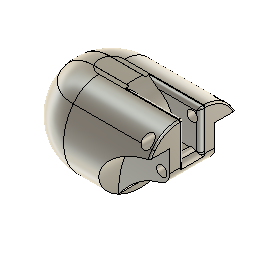
piece_4 (Autodesk Fusion 360 design; units mm, degrees)
Autodesk Fusion 360 part; units mm, degrees
sketch "Esboço1" plane through (0, 0, 0) normal (1, 0, 0) x (0, 1, 0)
  circle A0 centre (0, 0) radius 15
  dimension "d1" = 30
  constraint coincident A0.centre origin
  measures "d1" diameter of A0
extrude "Extrusão1" add sketch "Esboço1" along normal blind 40 makes body 1
fillet "Arredondamento1" radius 15 1 faces at (0, 3.8315, 5.6199) on bodies 1
sketch "Esboço2" plane through (40, 0, 0) normal (1, 0, 0) x (0, 1, 0)
  circle A0 centre (0, 0) radius 15
  line L0 (7.5, -12.9904) -> (-7.5, -12.9904)
  line L1 (-7.5, -12.9904) -> (-7.5, -7.9904)
  line L2 (-7.5, -7.9904) -> (7.5, -7.9904)
  line L3 (7.5, -7.9904) -> (7.5, -12.9904)
  line L4 (-7.5, -7.9904) -> (-15, -7.9904)
  line L5 (-15, -7.9904) -> (-15, -12.9904)
  line L6 (-15, -12.9904) -> (-7.5, -12.9904)
  line L7 (7.5, -7.9904) -> (15, -7.9904)
  line L8 (15, -7.9904) -> (15, -12.9904)
  line L9 (15, -12.9904) -> (7.5, -12.9904)
  dimension "d6" = 15
  dimension "d7" = 5
  dimension "d8" = 15
  constraint coincident A0 L0.start
  constraint coincident A0 L0.end
  constraint horizontal L0
  constraint perpendicular L0 L1
  constraint perpendicular L1 L2
  constraint perpendicular L1 L4
  constraint perpendicular L4 L5
  constraint perpendicular L1 L6
  constraint perpendicular L3 L7
  constraint perpendicular L2 L8
  constraint perpendicular L3 L9
  measures "d6" distance of L0.start L0.end
  measures "d7" distance of L0.end L1.end
  measures "d8" distance of L1.end L2.end
extrude "Extrusão2" cut sketch "Esboço2" against normal blind 5 contours A0 L1 L4 | A0 L3 L7 bodies 1
ref_plane "Plano de trabalho1" through (0, -16, 0) normal (0, 1, 0) x (0, 0, 1)
sketch "Esboço3" plane through (0, -16, 0) normal (0, 1, 0) x (1, 0, 0)
  spline S0 degree 5 poles (16, 15) (15.9441, 13.8206) (15.8879, 11.5162) (15.9712, 8.2226) (16.4224, 4.1625) (17.5919, -0.3229) (19.4201, -4.1668) (21.9593, -7.3182) (25.2357, -9.7517) (29.217, -11.4985) (33.8488, -12.6118) (38.0314, -13.0377) (41.4196, -13.1125) (43.7882, -13.0553) (45, -13) knots 0 0 0 0 0 0 0.1 0.2 0.3 0.4 0.5 0.6 0.7 0.8 0.9 1 1 1 1 1 1
  line L0 (16, 15) -> (45, 15)
  line L1 (45, 15) -> (45, -13)
  point P0 (22, -7)
  constraint horizontal L0
  constraint perpendicular L0 L1
extrude "Extrusão3" cut sketch "Esboço3" along normal blind 9 bodies 1
mirror "Espelhar1" about plane through (0, 0, 0) normal (0, 1, 0) of "Extrusão3"
sketch "Esboço4" plane through (0, -7, 0) normal (0, -1, 0) x (1, 0, 0)
  line L0 (15.9414, -13.2665) -> (40, -13.2665)
  spline S0 degree 5 poles (15.9414, -13.2665) (15.9255, -12.4614) (15.9203, -10.5419) (16.0411, -7.6201) (16.4922, -3.8951) (17.5919, 0.3229) (19.4201, 4.1668) (21.9593, 7.3182) (25.2357, 9.7517) (29.217, 11.4985) (33.0533, 12.4206) (36.2575, 12.8334) (38.5721, 12.9877) (39.8423, 13.0344) (40, 13.0397) knots 0.029806 0.029806 0.029806 0.029806 0.029806 0.029806 0.1 0.2 0.3 0.4 0.5 0.6 0.7 0.8 0.9 0.914124 0.914124 0.914124 0.914124 0.914124 0.914124
  circle A0 centre (37.5, -10.2665) radius 1.6
  line L1 (40, -13.2665) -> (40, 13.0397)
  dimension "d16" = 3.2
  dimension "d18" = 3
  dimension "d53" = 2.5
  measures "d16" diameter of A0
  measures "d18" distance of L0 A0.centre
  measures "d53" distance of A0.centre L1
extrude "Extrusão4" cut sketch "Esboço4" against normal blind 14 contours A0 bodies 1
sketch "Esboço5" plane through (40, 0, 0) normal (1, 0, 0) x (0, 1, 0)
  arc A0 (7.4139, 13.0397) -> (-7.4139, 13.0397) centre (0, 0) ccw
  line L0 (-2.5, 14.7902) -> (2.5, 14.7902)
  line L1 (2.5, 14.7902) -> (2.5, 1)
  line L2 (2.5, 1) -> (-2.5, 1)
  line L3 (-2.5, 1) -> (-2.5, 14.7902)
  line L4 (7, -13.2665) -> (7, 13.0397)
  line L5 (7, 13.0397) -> (7.4139, 13.0397)
  line L6 (-7.4139, 13.0397) -> (-7, 13.0397)
  line L7 (-7, 13.0397) -> (-7, -13.2665)
  arc A1 (-7, -13.2665) -> (7, -13.2665) centre (0, 0) ccw
  dimension "d21" = 5
  dimension "d22" = 2.5
  constraint horizontal L0
  constraint vertical L1
  constraint horizontal L2
  constraint vertical L3
  constraint coincident A0 L0.start
  measures "d21" distance of L0.start L0.end
  measures "d22" distance of A0.centre L3
extrude "Extrusão5" cut sketch "Esboço5" against normal blind 8 contours A0 L0 | L0 L1 L2 L3 bodies 1
sketch "Esboço6" plane through (0, 2.5, 0) normal (0, -1, 0) x (1, 0, 0)
  line L0 (40, 1) -> (40, 14.7902)
  line L1 (40, 14.7902) -> (32, 14.7902)
  line L2 (32, 14.7902) -> (32, 1)
  line L3 (32, 1) -> (40, 1)
  circle A0 centre (37.5, 9.7342) radius 1.6
  dimension "d25" = 3.2
  dimension "d26" = 2.5
  dimension "d27" = 5.056
  measures "d25" diameter of A0
  measures "d26" distance of L0 A0.centre
  measures "d27" distance of L1 A0.centre
extrude "Extrusão6" cut sketch "Esboço6" against normal blind 14 contours A0 bodies 1
extrude "Extrusão7" cut sketch "Esboço6" along normal blind 22 contours A0 bodies 1
copy_body "Corpo -> Componente1" bodies 1 removing the originals makes body 2 in component "Component'"
sketch "Esboço7" plane through (40, 0, 0) normal (1, 0, 0) x (0, 1, 0)
  line L0 (2.5, 14.7902) -> (2.5, 1)
  line L1 (2.5, 1) -> (-2.5, 1)
  line L2 (-2.5, 1) -> (-2.5, 14.7902)
  arc A0 (-2.5, 14.7902) -> (-7.4139, 13.0397) centre (0, 0) ccw
  line L3 (-7.4139, 13.0397) -> (-7, 13.0397)
  line L4 (-7, 13.0397) -> (-7, -13.2665)
  arc A1 (-7, -13.2665) -> (7, -13.2665) centre (0, 0) ccw
  line L5 (7, -13.2665) -> (7, 13.0397)
  line L6 (7, 13.0397) -> (7.4139, 13.0397)
  arc A2 (7.4139, 13.0397) -> (2.5, 14.7902) centre (0, 0) ccw
  line L7 (-7.4139, 13.0397) -> (7.4139, 13.0397)
  constraint coincident A0.end L3.start
  constraint coincident L6.end A2.start
extrude "Extrusão1'" cut sketch "Esboço7" against normal blind 8 contours L0 L6 A2 L7 | L2 A0 L3 L7 bodies 2 in component "Component'"
sketch "Esboço8" plane through (32, 0, 0) normal (1, 0, 0) x (0, 1, 0)
  arc A0 (7.4139, 13.0397) -> (-7.4139, 13.0397) centre (0, 0) ccw
  line L0 (-7.4139, 13.0397) -> (-2.5, 13.0397)
  line L1 (-2.5, 13.0397) -> (-2.5, 1)
  line L2 (-2.5, 1) -> (2.5, 1)
  line L3 (2.5, 1) -> (2.5, 13.0397)
  line L4 (2.5, 13.0397) -> (7.4139, 13.0397)
  line L5 (-2.5, 13.0397) -> (2.5, 13.0397)
  constraint coincident L0.end L1.start
  constraint coincident L3.end L4.start
fillet "Arredondamento5" radius 2 1 edges at (40, 0, 1) on bodies 2 in component "Component'"
sketch "Esboço9" plane through (0, -7, 0) normal (0, -1, 0) x (1, 0, 0)
  circle A0 centre (37.5, -10.2665) radius 1.6
  circle A1 centre (37.5, 9.7342) radius 1.6
  spline S0 degree 5 poles (15.9414, -13.2665) (15.9255, -12.4614) (15.9203, -10.5419) (16.0411, -7.6201) (16.4922, -3.8951) (17.5919, 0.3229) (19.4201, 4.1668) (21.9593, 7.3182) (25.2357, 9.7517) (29.217, 11.4985) (33.0533, 12.4206) (36.2575, 12.8334) (38.5721, 12.9877) (39.8423, 13.0344) (40, 13.0397) knots 0.029806 0.029806 0.029806 0.029806 0.029806 0.029806 0.1 0.2 0.3 0.4 0.5 0.6 0.7 0.8 0.9 0.914124 0.914124 0.914124 0.914124 0.914124 0.914124
  line L0 (15.9414, -13.2665) -> (40, -13.2665)
  spline S1 degree 5 poles (15.9414, -13.2665) (15.9568, -12.2565) (16.028, -10.2751) (16.2558, -7.4185) (16.8058, -3.8447) (17.9316, 0.204) (19.536, 3.7958) (21.6598, 6.8918) (24.3281, 9.4678) (27.5235, 11.5408) (31.2077, 13.147) (34.5148, 14.0885) (37.1849, 14.6135) (39.0478, 14.8844) (40, 15) knots 0 0 0 0 0 0 0.1 0.2 0.3 0.4 0.5 0.6 0.7 0.8 0.9 1 1 1 1 1 1
  line L1 (40, 15) -> (40, -13.2665)
  line L2 (40, -13.2665) -> (15.9414, -13.2665)
  line L3 (40, -13.2665) -> (40, 13.0397)
  point P0 (22, 7)
  constraint coincident S0.start L0.start
  constraint coincident S0 P0
  constraint perpendicular L0 L1
  constraint perpendicular L1 L2
extrude "Extrusão3'" cut sketch "Esboço9" along normal blind 14 contours S0 L0 S1 L1 L2 L3 | S0 S1 L1 bodies 2 in component "Component'"
mirror "Espelhar1'" about plane through (0, 0, 0) normal (0, 1, 0) of "Extrusão3'" in component "Component'"
sketch "Esboço10" plane through (0, -7, 0) normal (0, -1, 0) x (1, 0, 0)
  circle A0 centre (37.5, 9.7342) radius 1.6
  circle A1 centre (37.5, -10.2665) radius 1.6
  spline S0 degree 5 poles (15.9414, -13.2665) (15.9255, -12.4614) (15.9203, -10.5419) (16.0411, -7.6201) (16.4922, -3.8951) (17.5804, 0.2785) (19.0183, 3.3218) (20.4014, 5.2937) (21.4541, 6.4625) (22, 7) knots 0.029806 0.029806 0.029806 0.029806 0.029806 0.029806 0.1 0.2 0.3 0.4 0.495047 0.495047 0.495047 0.495047 0.495047 0.495047
  line L0 (15.9414, -13.2665) -> (40, -13.2665)
  spline S1 degree 5 poles (22, 7) (22.4471, 7.5113) (23.4297, 8.536) (25.0754, 9.9523) (27.0517, 11.2242) (29.2603, 12.2744) (30.9211, 12.9094) (31.8461, 13.2223) (31.9791, 13.2665) knots 0.508452 0.508452 0.508452 0.508452 0.508452 0.508452 0.6 0.7 0.8 0.816707 0.816707 0.816707 0.816707 0.816707 0.816707
  spline S2 degree 5 poles (33, -16) (32.9845, -15.3571) (32.9747, -14.0983) (33.0237, -12.2917) (33.2186, -10.0487) (33.6935, -7.5407) (34.4229, -5.3583) (35.4317, -3.5334) (36.7405, -2.0922) (38.3487, -1.034) (40.2384, -0.336) (41.9594, -0.0452) (43.3607, 0.0315) (44.3432, 0.0208) (44.8465, 0) knots 0 0 0 0 0 0 0.1 0.2 0.3 0.4 0.5 0.6 0.7 0.8 0.9 1 1 1 1 1 1
  line L1 (33, -16) -> (44.8465, -16)
  line L2 (44.8465, -16) -> (44.8465, 0)
  line L3 (40, -13.2665) -> (40, 13.0397)
  line L4 (40, 13.0397) -> (32, 13.0397)
  line L5 (32, 13.0397) -> (32, 13.2665)
  line L6 (32, 13.2665) -> (31.9791, 13.2665)
  point P0 (36, -3)
  constraint perpendicular L1 L2
sketch "Esboço11" plane through (40, 0, 0) normal (1, 0, 0) x (0, 1, 0)
  line L0 (-2.5, -1) -> (-2.5, 13.0397)
  line L1 (-2.5, 13.0397) -> (-7, 13.0397)
  line L2 (-7, 13.0397) -> (-7, -13.2665)
  arc A0 (-7, -13.2665) -> (7, -13.2665) centre (0, 0) ccw
  line L3 (7, -13.2665) -> (7, 13.0397)
  line L4 (2.5, 13.0397) -> (2.5, -1)
  line L5 (2.5, -1) -> (-2.5, -1)
  circle A1 centre (0, 0) radius 15
  line L6 (7, 13.0397) -> (2.5, 13.0397)
  line L7 (-2.5, 13.0397) -> (2.5, 13.0397)
  dimension "d62" = 30
  constraint concentric A0 A1
  constraint coincident L0.end L1.start
  constraint coincident L4.start L6.end
  measures "d62" diameter of A1
extrude "Extrusão5'" add sketch "Esboço11" against normal blind 25 contours L1 L2 L3 A1 L6 L7 bodies 2 in component "Component'"
sketch "Esboço12" plane through (0, -16, 0) normal (0, 1, 0) x (1, 0, 0)
  spline S0 degree 5 poles (24, 15) (23.9922, 14.2256) (24.0046, 12.7054) (24.1071, 10.5108) (24.4146, 7.7588) (25.1035, 4.6295) (26.1261, 1.8405) (27.5131, -0.5768) (29.2866, -2.5998) (31.4398, -4.2355) (33.9474, -5.5097) (36.2155, -6.2618) (38.0549, -6.6849) (39.3415, -6.9052) (40, -7) knots 0 0 0 0 0 0 0.1 0.2 0.3 0.4 0.5 0.6 0.7 0.8 0.9 1 1 1 1 1 1
  line L0 (24, 15) -> (40, 15)
  line L1 (40, 15) -> (40, -7)
  point P0 (28, -1)
  constraint horizontal L0
  constraint perpendicular L0 L1
extrude "Extrusão6'" cut sketch "Esboço12" along normal blind 9 bodies 2 in component "Component'"
mirror "Espelhar2" about plane through (0, 0, 0) normal (0, 1, 0) of "Extrusão6'" in component "Component'"
sketch "Esboço13" plane through (40, 0, 0) normal (1, 0, 0) x (0, 1, 0)
  line L0 (7, 7) -> (13.2665, 7)
  arc A0 (13.2665, 7) -> (-13.2665, 7) centre (0, 0) ccw
  line L1 (-13.2665, 7) -> (-7, 7)
  line L2 (-7, 7) -> (-7, -13.2665)
  arc A1 (-7, -13.2665) -> (7, -13.2665) centre (0, 0) ccw
  line L3 (7, -13.2665) -> (7, 7)
  line L4 (2.5, 13.0397) -> (2.5, -1)
  line L5 (2.5, -1) -> (-2.5, -1)
  line L6 (-2.5, -1) -> (-2.5, 13.0397)
  line L7 (-2.5, 13.0397) -> (2.5, 13.0397)
  line L8 (-13, 13) -> (19, 13)
  line L9 (19, 13) -> (19, 23)
  line L10 (19, 23) -> (-13, 23)
  line L11 (-13, 23) -> (-13, 13)
  constraint horizontal L8
  constraint perpendicular L8 L9
  constraint perpendicular L9 L10
  constraint perpendicular L8 L11
extrude "Extrusão7'" cut sketch "Esboço13" against normal blind 52 contours A0 L4 L6 L7 L8 bodies 2 in component "Component'"
extrude "Extrusão8" cut 1 faces at (37.3813, 7, 10.138) along direction (0, 1, 0) blind 6 on bodies 2 bodies 2 in component "Component'"
extrude "Extrusão9" cut 1 faces at (38.5193, -7, 10.0486) along direction (0, -1, 0) blind 6.5 on bodies 2 bodies 2 in component "Component'"
fillet "Arredondamento10" radius 10 5 edges at (10.6819, 6.1118, 13) (27.5, 7.4833, 13) (7.5861, 0, 13.0397) (27.5, -7.4833, 13) (10.6819, -6.1118, 13) on bodies 2 in component "Component'"
fillet "Arredondamento11" radius 10 1 edges at (32, 0, 13.0397) on bodies 2 in component "Component'"
fillet "Arredondamento12" radius 0.5 6 edges at (40, -3.25, 13) (40, -8.4721, 11.9443) (40, -12.6728, 8.025) (40, 12.6728, 8.025) (40, 8.4721, 11.9443) (40, 3.25, 13) on bodies 2 in component "Component'"
sketch "Esboço14" plane through (0, -7, 0) normal (0, -1, 0) x (1, 0, 0)
  line L0 (24.0113, -13.2665) -> (40, -13.2665)
  line L1 (40, -13.2665) -> (40, 7)
  spline S0 degree 5 poles (24.0113, -13.2665) (24.0209, -12.8589) (24.0601, -11.7151) (24.1803, -9.8874) (24.4774, -7.4738) (25.1035, -4.6295) (26.1261, -1.8405) (27.5131, 0.5768) (29.2866, 2.5998) (31.4398, 4.2355) (33.9474, 5.5097) (36.2155, 6.2618) (38.0549, 6.6849) (39.3415, 6.9052) (40, 7) knots 0.045537 0.045537 0.045537 0.045537 0.045537 0.045537 0.1 0.2 0.3 0.4 0.5 0.6 0.7 0.8 0.9 1 1 1 1 1 1
  circle A0 centre (37.5, -10.2665) radius 1.6
  circle A1 centre (37.5, -0.2665) radius 1.6
  dimension "d83" = 3.2
  dimension "d84" = 10
  measures "d83" diameter of A1
  measures "d84" distance of A0.centre A1.centre
extrude "Extrusão10" cut sketch "Esboço14" against normal blind 17 contours A1 bodies 2 in component "Component'"
sketch "Esboço15" plane through (0, -7, 0) normal (0, -1, 0) x (1, 0, 0)
  circle A0 centre (37.5, -0.2665) radius 1.6
  line L0 (24.0113, -13.2665) -> (40, -13.2665)
  line L1 (40, -13.2665) -> (40, 7)
  spline S0 degree 5 poles (24.0113, -13.2665) (24.0209, -12.8589) (24.0601, -11.7151) (24.1803, -9.8874) (24.4774, -7.4738) (25.1035, -4.6295) (26.1261, -1.8405) (27.5131, 0.5768) (29.2866, 2.5998) (31.4398, 4.2355) (33.9474, 5.5097) (36.2155, 6.2618) (38.0549, 6.6849) (39.3415, 6.9052) (40, 7) knots 0.045537 0.045537 0.045537 0.045537 0.045537 0.045537 0.1 0.2 0.3 0.4 0.5 0.6 0.7 0.8 0.9 1 1 1 1 1 1
  circle A1 centre (37.5, -10.2665) radius 1.6
  line L2 (24.0113, -18.0539) -> (41, -18.0539)
  line L3 (41, -18.0539) -> (41, -3)
  line L4 (24.0113, -18.0539) -> (24.0113, -13.2665)
  spline S1 degree 5 poles (24.0113, -13.2665) (24.2992, -12.8891) (24.8794, -12.149) (25.763, -11.0831) (26.9683, -9.7516) (28.5231, -8.2472) (30.1308, -6.9182) (31.7962, -5.7804) (33.5227, -4.8454) (35.3092, -4.1093) (37.1516, -3.5586) (38.6668, -3.2552) (39.8251, -3.0999) (40.6068, -3.028) (41, -3) knots 0 0 0 0 0 0 0.1 0.2 0.3 0.4 0.5 0.6 0.7 0.8 0.9 1 1 1 1 1 1
  point P0 (32.1946, -5.6029)
  constraint parallel L0 L2
  constraint perpendicular L2 L3
  constraint coincident L0.start S0.start
  constraint perpendicular L0 L4
extrude "Extrusão11" cut sketch "Esboço15" against normal blind 30 contours L0 L1 S1 | L0 L1 L2 L3 L4 S1 bodies 2 in component "Component'"
fillet "Arredondamento14" radius 4 1 edges at (40, 0, -3.0925) on bodies 2 in component "Component'"
scale "Escala1" factor 0.7 about (35.9, -7, -0.2665) bodies 2 in component "Component'"
scale "Escala2" factor 1.14 about (27.5779, -7, -9.3665) bodies 2 in component "Component'"
fillet "Arredondamento15" radius 1 8 edges at (33.3105, 0.581, 11.5942) (40.22, 0.581, 11.4773) (40.3369, 0.581, 6.2993) (40.3238, 0.581, 1.1143) (40.3238, -3.409, 1.1143) (40.3369, -3.409, 6.2993) (40.22, -3.409, 11.4773) (33.3105, -3.409, 11.5942) on bodies 2 in component "Component'"
component "Component'" placed x (1, 0, 0) y (0, 1, 0) z (0, 0, 1) at (0, 0, 0)
